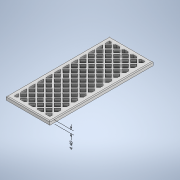
# Autodesk Inventor part: Part_B3
Saved by Autodesk Inventor 2022.6 (Build 266554010, 554A)
## iProperties
Created: 2025-05-15
Part Number: Part_B3
Material: Generic
Document SubType Name: Modeling
Designer: khinm
Density: 1 g/cm^3
Appearance: Default
Author: khinm
Autodesk Inventor part; units mm, degrees
ref_plane "YZ Plane" through (0, 0, 0) normal (1, 0, 0) x (0, 1, 0)
ref_plane "XZ Plane" through (0, 0, 0) normal (0, 1, 0) x (-1, 0, 0)
ref_plane "XY Plane" through (0, 0, 0) normal (0, 0, 1) x (1, 0, 0)
sketch "Sketch1" plane through (0, 0, 0) normal (0, 1, 0) x (-1, 0, 0)
  line L0 (27.35, -64.7) -> (-27.35, -64.7)
  line L1 (-27.35, -64.7) -> (-27.35, 64.7)
  line L2 (-27.35, 64.7) -> (27.35, 64.7)
  line L3 (27.35, 64.7) -> (27.35, -64.7)
  point P0 (0, 0)
  point P1 (27.35, 0)
  point P2 (0, -64.7)
  dimension "d0" = 54.7
  dimension "d1" = 129.4
  constraints: 8 end point, 2 midpoint, 2 parallel, 1 horizontal, 1 horizontal alignment, 1 perpendicular, 1 vertical alignment
  measures "d0" distance of L1.end L2.end
  measures "d1" distance between parallel lines of L2 L0
extrude "Extrusion1" add sketch "Sketch1" along normal mid plane 4.4
sketch "Sketch2" plane through (0, 2.2, 0) normal (0, 1, 0) x (1, 0, 0)
  line L0 (22.35, 59.7) -> (-22.35, 59.7)
  line L1 (-22.35, 59.7) -> (-22.35, -59.7)
  line L2 (-22.35, -59.7) -> (22.35, -59.7)
  line L3 (22.35, -59.7) -> (22.35, 59.7)
  line L4 (-27.35, -64.7) -> (27.35, -64.7) projected
  line L5 (-27.35, 64.7) -> (-27.35, -64.7) projected
  line L6 (-18.9137, 58.1363) -> (-22.35, 54.7)
  line L7 (21.949, -59.7) -> (22.35, -59.399)
  line L8 (-18.9137, -58.1363) -> (-22.35, -54.7)
  line L9 (21.899, 59.9) -> (22.4, 59.399)
  line L10 (16.3916, 58.1363) -> (19.8022, 54.7258)
  line L11 (21.6449, 53.033) -> (22.35, 52.328)
  line L12 (19.8772, 51.2652) -> (22.35, 48.7924)
  line L13 (22.35, 53.7381) -> (21.6449, 53.033)
  line L14 (17.9553, 59.7) -> (16.3916, 58.1363)
  line L15 (11.2924, 59.7) -> (12.8561, 58.1363)
  line L16 (14.6239, 56.5685) -> (18.1594, 53.033)
  line L17 (12.8561, 58.1363) -> (9.3206, 54.6008)
  line L18 (5.785, 58.1363) -> (9.3206, 54.6008)
  line L19 (14.6239, 56.5685) -> (11.0883, 53.033)
  line L20 (11.0883, 53.033) -> (14.6239, 49.4975)
  line L21 (9.3206, 51.2652) -> (12.8561, 47.7297)
  line L22 (19.8772, 51.2652) -> (16.3416, 47.7297)
  line L23 (16.3416, 47.7297) -> (19.8772, 44.1942)
  line L24 (21.6449, 42.4264) -> (22.35, 41.7214)
  line L25 (14.6239, 45.9619) -> (18.1594, 42.4264)
  line L26 (19.8772, 40.6586) -> (22.35, 38.1858)
  line L27 (22.35, 46.667) -> (19.8772, 44.1942)
  line L28 (22.35, 43.1315) -> (21.6449, 42.4264)
  line L29 (19.8772, 40.6586) -> (16.3416, 37.1231)
  line L30 (18.1594, 42.4264) -> (14.6239, 38.8909)
  line L31 (14.6239, 45.9619) -> (11.0883, 42.4264)
  line L32 (11.0883, 42.4264) -> (14.6239, 38.8909)
  line L33 (12.8561, 37.1231) -> (9.3206, 40.6586)
  line L34 (12.8561, 47.7297) -> (9.3206, 44.1942)
  line L35 (5.785, 47.7297) -> (9.3206, 44.1942)
  line L36 (9.3206, 51.2652) -> (5.785, 47.7297)
  line L37 (7.5528, 42.4264) -> (4.0173, 45.9619)
  line L38 (7.5528, 53.033) -> (4.0173, 49.4975)
  line L39 (16.3416, 37.1231) -> (19.8772, 33.5876)
  line L40 (21.6449, 31.8198) -> (22.35, 31.1148)
  line L41 (22.35, 27.5792) -> (19.8772, 30.052)
  line L42 (18.1594, 31.8198) -> (14.6239, 35.3553)
  line L43 (22.35, 32.5249) -> (21.6449, 31.8198)
  line L44 (22.35, 36.0604) -> (19.8772, 33.5876)
  line L45 (22.35, 20.5082) -> (21.6449, 21.2132)
  line L46 (22.35, 16.9726) -> (19.8772, 19.4454)
  line L47 (22.35, 21.9183) -> (21.6449, 21.2132)
  line L48 (22.35, 25.4538) -> (19.8772, 22.981)
  line L49 (19.8772, 30.052) -> (16.3416, 26.5165)
  line L50 (19.8772, 22.981) -> (16.3416, 26.5165)
  line L51 (18.1594, 21.2132) -> (14.6239, 24.7487)
  line L52 (18.1594, 31.8198) -> (14.6239, 28.2843)
  line L53 (14.6239, 35.3553) -> (11.0883, 31.8198)
  line L54 (12.8561, 37.1231) -> (9.3206, 33.5876)
  line L55 (9.3206, 40.6586) -> (5.785, 37.1231)
  line L56 (7.5528, 42.4264) -> (4.0173, 38.8909)
  line L57 (14.6239, 28.2843) -> (11.0883, 31.8198)
  line L58 (12.8561, 26.5165) -> (9.3206, 30.052)
  line L59 (9.3206, 22.981) -> (5.785, 26.5165)
  line L60 (7.5528, 21.2132) -> (4.0173, 24.7487)
  line L61 (14.6239, 17.6777) -> (11.0883, 21.2132)
  line L62 (12.8561, 15.9099) -> (9.3206, 19.4454)
  line L63 (9.3206, 12.3744) -> (5.785, 15.9099)
  line L64 (7.5528, 10.6066) -> (4.0173, 14.1421)
  line L65 (22.35, 9.9016) -> (21.6449, 10.6066)
  line L66 (19.8772, 12.3744) -> (16.3416, 15.9099)
  line L67 (22.35, 6.366) -> (19.8772, 8.8388)
  line L68 (18.1594, 10.6066) -> (14.6239, 14.1421)
  line L69 (14.6239, 7.0711) -> (11.0883, 10.6066)
  line L70 (12.8561, 5.3033) -> (9.3206, 8.8388)
  line L71 (22.35, 11.3117) -> (21.6449, 10.6066)
  line L72 (22.35, 14.8472) -> (19.8772, 12.3744)
  line L73 (19.8772, 19.4454) -> (16.3416, 15.9099)
  line L74 (18.1594, 21.2132) -> (14.6239, 17.6777)
  line L75 (14.6239, 24.7487) -> (11.0883, 21.2132)
  line L76 (12.8561, 26.5165) -> (9.3206, 22.981)
  line L77 (9.3206, 30.052) -> (5.785, 26.5165)
  line L78 (7.5528, 31.8198) -> (4.0173, 28.2843)
  line L79 (-18.9137, 58.1363) -> (-20.4774, 59.7)
  line L80 (-8.3571, 58.1363) -> (-9.9208, 59.7)
  line L81 (-11.8926, 54.6008) -> (-15.4282, 58.1363)
  line L82 (-13.6604, 53.033) -> (-17.1959, 56.5685)
  line L83 (-17.1959, 49.4975) -> (-20.7315, 53.033)
  line L84 (-18.9137, 47.5297) -> (-22.35, 50.966)
  line L85 (-3.2579, 59.7) -> (-4.8216, 58.1363)
  line L86 (-6.5893, 56.5685) -> (-10.1249, 53.033)
  line L87 (-8.3571, 58.1363) -> (-11.8926, 54.6008)
  line L88 (-13.8645, 59.7) -> (-15.4282, 58.1363)
  line L89 (-17.1959, 56.5685) -> (-20.7315, 53.033)
  line L90 (-11.8926, 51.2652) -> (-15.4282, 47.7297)
  line L91 (-17.1959, 45.9619) -> (-20.7315, 42.4264)
  line L92 (-13.6604, 53.033) -> (-17.1959, 49.4975)
  line L93 (-18.9137, 47.5297) -> (-22.35, 44.0934)
  line L94 (0.6858, 59.7) -> (2.2495, 58.1363)
  line L95 (4.0173, 56.5685) -> (7.5528, 53.033)
  line L96 (-4.8216, 58.1363) -> (-1.286, 54.6008)
  line L97 (0.4817, 53.033) -> (4.0173, 49.4975)
  line L98 (2.2495, 47.7297) -> (-1.286, 51.2652)
  line L99 (-3.0538, 53.033) -> (-6.5893, 56.5685)
  line L100 (-6.5893, 49.4975) -> (-10.1249, 53.033)
  line L101 (-8.3571, 47.7297) -> (-11.8926, 51.2652)
  line L102 (-11.8926, 44.1942) -> (-15.4282, 47.7297)
  line L103 (-13.6604, 42.4264) -> (-17.1959, 45.9619)
  line L104 (-17.1959, 38.8909) -> (-20.7315, 42.4264)
  line L105 (-18.9137, 36.9231) -> (-22.35, 40.3594)
  line L106 (7.3487, 59.7) -> (5.785, 58.1363)
  line L107 (4.0173, 56.5685) -> (0.4817, 53.033)
  line L108 (2.2495, 58.1363) -> (-1.286, 54.6008)
  line L109 (4.0173, 45.9619) -> (0.4817, 42.4264)
  line L110 (2.2495, 47.7297) -> (-1.286, 44.1942)
  line L111 (-1.286, 51.2652) -> (-4.8216, 47.7297)
  line L112 (-3.0538, 53.033) -> (-6.5893, 49.4975)
  line L113 (-1.286, 40.6586) -> (-4.8216, 37.1231)
  line L114 (-3.0538, 42.4264) -> (-6.5893, 38.8909)
  line L115 (-6.5893, 45.9619) -> (-10.1249, 42.4264)
  line L116 (-8.3571, 47.7297) -> (-11.8926, 44.1942)
  line L117 (-6.5893, 35.3553) -> (-10.1249, 31.8198)
  line L118 (-8.3571, 37.1231) -> (-11.8926, 33.5876)
  line L119 (-11.8926, 40.6586) -> (-15.4282, 37.1231)
  line L120 (-17.1959, 35.3553) -> (-20.7315, 31.8198)
  line L121 (-13.6604, 42.4264) -> (-17.1959, 38.8909)
  line L122 (-18.9137, 36.9231) -> (-22.35, 33.4868)
  line L123 (-11.8926, 30.052) -> (-15.4282, 26.5165)
  line L124 (-17.1959, 24.7487) -> (-20.7315, 21.2132)
  line L125 (-13.6604, 31.8198) -> (-17.1959, 28.2843)
  line L126 (-18.9137, 26.3165) -> (-22.35, 22.8802)
  line L127 (9.3206, 33.5876) -> (5.785, 37.1231)
  line L128 (7.5528, 31.8198) -> (4.0173, 35.3553)
  line L129 (4.0173, 28.2843) -> (0.4817, 31.8198)
  line L130 (2.2495, 26.5165) -> (-1.286, 30.052)
  line L131 (-17.1959, 17.6777) -> (-20.7315, 21.2132)
  line L132 (-18.9137, 15.7099) -> (-22.35, 19.1462)
  line L133 (4.0173, 35.3553) -> (0.4817, 31.8198)
  line L134 (2.2495, 37.1231) -> (-1.286, 33.5876)
  line L135 (-1.286, 30.052) -> (-4.8216, 26.5165)
  line L136 (-3.0538, 31.8198) -> (-6.5893, 28.2843)
  line L137 (-6.5893, 24.7487) -> (-10.1249, 21.2132)
  line L138 (-8.3571, 26.5165) -> (-11.8926, 22.981)
  line L139 (-11.8926, 19.4454) -> (-15.4282, 15.9099)
  line L140 (-17.1959, 14.1421) -> (-20.7315, 10.6066)
  line L141 (-13.6604, 21.2132) -> (-17.1959, 17.6777)
  line L142 (-18.9137, 15.7099) -> (-22.35, 12.2736)
  line L143 (4.0173, 17.6777) -> (0.4817, 21.2132)
  line L144 (-1.286, 22.981) -> (-4.8216, 26.5165)
  line L145 (2.2495, 15.9099) -> (-1.286, 19.4454)
  line L146 (-3.0538, 21.2132) -> (-6.5893, 24.7487)
  line L147 (-6.5893, 17.6777) -> (-10.1249, 21.2132)
  line L148 (-8.3571, 15.9099) -> (-11.8926, 19.4454)
  line L149 (-11.8926, 12.3744) -> (-15.4282, 15.9099)
  line L150 (-13.6604, 10.6066) -> (-17.1959, 14.1421)
  line L151 (-17.1959, 7.0711) -> (-20.7315, 10.6066)
  line L152 (-18.9137, 5.1033) -> (-22.35, 8.5396)
  line L153 (4.0173, 7.0711) -> (0.4817, 10.6066)
  line L154 (-1.286, 12.3744) -> (-4.8216, 15.9099)
  line L155 (2.2495, 5.3033) -> (-1.286, 8.8388)
  line L156 (-3.0538, 10.6066) -> (-6.5893, 14.1421)
  line L157 (-6.5893, 7.0711) -> (-10.1249, 10.6066)
  line L158 (-8.3571, 5.3033) -> (-11.8926, 8.8388)
  line L159 (-11.8926, 1.7678) -> (-15.4282, 5.3033)
  line L160 (-13.6604, 0) -> (-17.1959, 3.5355)
  line L161 (-17.1959, -3.5355) -> (-20.7315, 0)
  line L162 (-18.9137, -5.5033) -> (-22.35, -2.067)
  line L163 (-1.286, 1.7678) -> (-4.8216, 5.3033)
  line L164 (-3.0538, 0) -> (-6.5893, 3.5355)
  line L165 (-6.5893, -3.5355) -> (-10.1249, 0)
  line L166 (-8.3571, -5.3033) -> (-11.8926, -1.7678)
  line L167 (-11.8926, -8.8388) -> (-15.4282, -5.3033)
  line L168 (-13.6604, -10.6066) -> (-17.1959, -7.0711)
  line L169 (-17.1959, -14.1421) -> (-20.7315, -10.6066)
  line L170 (-18.9137, -16.1099) -> (-22.35, -12.6736)
  line L171 (9.3206, 1.7678) -> (5.785, 5.3033)
  line L172 (7.5528, 0) -> (4.0173, 3.5355)
  line L173 (4.0173, -3.5355) -> (0.4817, 0)
  line L174 (2.2495, -5.3033) -> (-1.286, -1.7678)
  line L175 (-1.286, -8.8388) -> (-4.8216, -5.3033)
  line L176 (-3.0538, -10.6066) -> (-6.5893, -7.0711)
  line L177 (-6.5893, -14.1421) -> (-10.1249, -10.6066)
  line L178 (-8.3571, -15.9099) -> (-11.8926, -12.3744)
  line L179 (-11.8926, -19.4454) -> (-15.4282, -15.9099)
  line L180 (-13.6604, -21.2132) -> (-17.1959, -17.6777)
  line L181 (-17.1959, -24.7487) -> (-20.7315, -21.2132)
  line L182 (-18.9137, -26.7165) -> (-22.35, -23.2802)
  line L183 (-18.9137, -37.3231) -> (-22.35, -33.8868)
  line L184 (-17.1959, -35.3553) -> (-20.7315, -31.8198)
  line L185 (-13.6604, -31.8198) -> (-17.1959, -28.2843)
  line L186 (-11.8926, -30.052) -> (-15.4282, -26.5165)
  line L187 (-8.3571, -26.5165) -> (-11.8926, -22.981)
  line L188 (-6.5893, -24.7487) -> (-10.1249, -21.2132)
  line L189 (-3.0538, -21.2132) -> (-6.5893, -17.6777)
  line L190 (-1.286, -19.4454) -> (-4.8216, -15.9099)
  line L191 (2.2495, -15.9099) -> (-1.286, -12.3744)
  line L192 (4.0173, -14.1421) -> (0.4817, -10.6066)
  line L193 (7.5528, -10.6066) -> (4.0173, -7.0711)
  line L194 (9.3206, -8.8388) -> (5.785, -5.3033)
  line L195 (22.35, -0.7051) -> (21.6449, 0)
  line L196 (19.8772, 1.7678) -> (16.3416, 5.3033)
  line L197 (22.35, 0) -> (21.6449, 0)
  line L198 (22.35, -4.2406) -> (19.8772, -1.7678)
  line L199 (18.1594, 0) -> (14.6239, 3.5355)
  line L200 (14.6239, -3.5355) -> (11.0883, 0)
  line L201 (12.8561, -5.3033) -> (9.3206, -1.7678)
  line L202 (22.35, -11.3117) -> (21.6449, -10.6066)
  line L203 (19.8772, -8.8388) -> (16.3416, -5.3033)
  line L204 (22.35, -14.8472) -> (19.8772, -12.3744)
  line L205 (18.1594, -10.6066) -> (14.6239, -7.0711)
  line L206 (14.6239, -14.1421) -> (11.0883, -10.6066)
  line L207 (12.8561, -15.9099) -> (9.3206, -12.3744)
  line L208 (9.3206, -19.4454) -> (5.785, -15.9099)
  line L209 (7.5528, -21.2132) -> (4.0173, -17.6777)
  line L210 (4.0173, -24.7487) -> (0.4817, -21.2132)
  line L211 (2.2495, -26.5165) -> (-1.286, -22.981)
  line L212 (-1.286, -30.052) -> (-4.8216, -26.5165)
  line L213 (-3.0538, -31.8198) -> (-6.5893, -28.2843)
  line L214 (-6.5893, -35.3553) -> (-10.1249, -31.8198)
  line L215 (-8.3571, -37.1231) -> (-11.8926, -33.5876)
  line L216 (-11.8926, -40.6586) -> (-15.4282, -37.1231)
  line L217 (-13.6604, -42.4264) -> (-17.1959, -38.8909)
  line L218 (-17.1959, -45.9619) -> (-20.7315, -42.4264)
  line L219 (-18.9137, -47.9297) -> (-22.35, -44.4934)
  line L220 (22.35, -21.9183) -> (21.6449, -21.2132)
  line L221 (19.8772, -19.4454) -> (16.3416, -15.9099)
  line L222 (22.35, -25.4538) -> (19.8772, -22.981)
  line L223 (18.1594, -21.2132) -> (14.6239, -17.6777)
  line L224 (14.6239, -24.7487) -> (11.0883, -21.2132)
  line L225 (12.8561, -26.5165) -> (9.3206, -22.981)
  line L226 (9.3206, -30.052) -> (5.785, -26.5165)
  line L227 (7.5528, -31.8198) -> (4.0173, -28.2843)
  line L228 (4.0173, -35.3553) -> (0.4817, -31.8198)
  line L229 (2.2495, -37.1231) -> (-1.286, -33.5876)
  line L230 (-1.286, -40.6586) -> (-4.8216, -37.1231)
  line L231 (-3.0538, -42.4264) -> (-6.5893, -38.8909)
  line L232 (-6.5893, -45.9619) -> (-10.1249, -42.4264)
  line L233 (-8.3571, -47.7297) -> (-11.8926, -44.1942)
  line L234 (-11.8926, -51.2652) -> (-15.4282, -47.7297)
  line L235 (-8.3071, -58.1363) -> (-11.8426, -54.6008)
  line L236 (-13.6604, -53.033) -> (-17.1959, -49.4975)
  line L237 (-13.8145, -59.7) -> (-15.3782, -58.1363)
  line L238 (-17.1959, -56.5685) -> (-20.7315, -53.033)
  line L239 (22.35, -32.5249) -> (21.6449, -31.8198)
  line L240 (19.8772, -30.052) -> (16.3416, -26.5165)
  line L241 (22.35, -36.0604) -> (19.8772, -33.5876)
  line L242 (18.1594, -31.8198) -> (14.6239, -28.2843)
  line L243 (14.6239, -35.3553) -> (11.0883, -31.8198)
  line L244 (12.8561, -37.1231) -> (9.3206, -33.5876)
  line L245 (9.3206, -40.6586) -> (5.785, -37.1231)
  line L246 (7.5528, -42.4264) -> (4.0173, -38.8909)
  line L247 (4.0173, -45.9619) -> (0.4817, -42.4264)
  line L248 (2.2495, -47.7297) -> (-1.286, -44.1942)
  line L249 (-1.286, -51.2652) -> (-4.8216, -47.7297)
  line L250 (2.2995, -58.1363) -> (-1.236, -54.6008)
  line L251 (-3.0538, -53.033) -> (-6.5893, -49.4975)
  line L252 (-3.2079, -59.7) -> (-4.7716, -58.1363)
  line L253 (-6.5893, -56.5685) -> (-10.1249, -53.033)
  line L254 (22.35, -43.1315) -> (21.6449, -42.4264)
  line L255 (19.8772, -40.6586) -> (16.3416, -37.1231)
  line L256 (22.35, -46.667) -> (19.8772, -44.1942)
  line L257 (18.1594, -42.4264) -> (14.6239, -38.8909)
  line L258 (14.6239, -45.9619) -> (11.0883, -42.4264)
  line L259 (12.8561, -47.7297) -> (9.3206, -44.1942)
  line L260 (9.3206, -51.2652) -> (5.785, -47.7297)
  line L261 (12.9061, -58.1363) -> (9.3706, -54.6008)
  line L262 (7.5528, -53.033) -> (4.0173, -49.4975)
  line L263 (7.3987, -59.7) -> (5.835, -58.1363)
  line L264 (4.0173, -56.5685) -> (0.4817, -53.033)
  line L265 (22.35, -53.7381) -> (21.6449, -53.033)
  line L266 (19.8772, -51.2652) -> (16.3416, -47.7297)
  line L267 (22.4, -57.2736) -> (19.9272, -54.8008)
  line L268 (18.1594, -53.033) -> (14.6239, -49.4975)
  line L269 (17.9553, -59.9) -> (16.3916, -58.3363)
  line L270 (14.6239, -56.5685) -> (11.0883, -53.033)
  line L271 (-18.9137, -58.1363) -> (-20.4774, -59.7)
  line L272 (-8.3071, -58.1363) -> (-9.8708, -59.7)
  line L273 (-11.8426, -54.6008) -> (-15.3782, -58.1363)
  line L274 (-13.6604, -53.033) -> (-17.1959, -56.5685)
  line L275 (-17.1959, -49.4975) -> (-20.7315, -53.033)
  line L276 (-18.9137, -47.9297) -> (-22.35, -51.366)
  line L277 (0.7358, -59.7) -> (2.2995, -58.1363)
  line L278 (-4.7716, -58.1363) -> (-1.236, -54.6008)
  line L279 (-3.0538, -53.033) -> (-6.5893, -56.5685)
  line L280 (-6.5893, -49.4975) -> (-10.1249, -53.033)
  line L281 (-8.3571, -47.7297) -> (-11.8926, -51.2652)
  line L282 (-11.8926, -44.1942) -> (-15.4282, -47.7297)
  line L283 (-13.6604, -42.4264) -> (-17.1959, -45.9619)
  line L284 (-17.1959, -38.8909) -> (-20.7315, -42.4264)
  line L285 (-18.9137, -37.3231) -> (-22.35, -40.7594)
  line L286 (11.3424, -59.7) -> (12.9061, -58.1363)
  line L287 (5.835, -58.1363) -> (9.3706, -54.6008)
  line L288 (4.0173, -56.5685) -> (7.5528, -53.033)
  line L289 (0.4817, -53.033) -> (4.0173, -49.4975)
  line L290 (2.2495, -47.7297) -> (-1.286, -51.2652)
  line L291 (-1.286, -44.1942) -> (-4.8216, -47.7297)
  line L292 (-3.0538, -42.4264) -> (-6.5893, -45.9619)
  line L293 (-6.5893, -38.8909) -> (-10.1249, -42.4264)
  line L294 (-8.3571, -37.1231) -> (-11.8926, -40.6586)
  line L295 (-11.8926, -33.5876) -> (-15.4282, -37.1231)
  line L296 (-13.6604, -31.8198) -> (-17.1959, -35.3553)
  line L297 (-17.1959, -28.2843) -> (-20.7315, -31.8198)
  line L298 (-18.9137, -26.7165) -> (-22.35, -30.1528)
  line L299 (-18.9137, -16.1099) -> (-22.35, -19.5462)
  line L300 (-17.1959, -17.6777) -> (-20.7315, -21.2132)
  line L301 (-13.6604, -21.2132) -> (-17.1959, -24.7487)
  line L302 (-11.8926, -22.981) -> (-15.4282, -26.5165)
  line L303 (-8.3571, -26.5165) -> (-11.8926, -30.052)
  line L304 (-6.5893, -28.2843) -> (-10.1249, -31.8198)
  line L305 (-3.0538, -31.8198) -> (-6.5893, -35.3553)
  line L306 (-1.286, -33.5876) -> (-4.8216, -37.1231)
  line L307 (2.2495, -37.1231) -> (-1.286, -40.6586)
  line L308 (4.0173, -38.8909) -> (0.4817, -42.4264)
  line L309 (7.5528, -42.4264) -> (4.0173, -45.9619)
  line L310 (5.785, -47.7297) -> (9.3206, -44.1942)
  line L311 (9.3206, -51.2652) -> (12.8561, -47.7297)
  line L312 (11.0883, -53.033) -> (14.6239, -49.4975)
  line L313 (14.6239, -56.5685) -> (18.1594, -53.033)
  line L314 (19.8772, -51.2652) -> (22.35, -48.7924)
  line L315 (16.3916, -58.3363) -> (19.9272, -54.8008)
  line L316 (21.6449, -53.033) -> (22.35, -52.328)
  line L317 (-18.9137, -5.5033) -> (-22.35, -8.9396)
  line L318 (-17.1959, -7.0711) -> (-20.7315, -10.6066)
  line L319 (-13.6604, -10.6066) -> (-17.1959, -14.1421)
  line L320 (-11.8926, -12.3744) -> (-15.4282, -15.9099)
  line L321 (-8.3571, -15.9099) -> (-11.8926, -19.4454)
  line L322 (-6.5893, -17.6777) -> (-10.1249, -21.2132)
  line L323 (-3.0538, -21.2132) -> (-6.5893, -24.7487)
  line L324 (-1.286, -22.981) -> (-4.8216, -26.5165)
  line L325 (2.2495, -26.5165) -> (-1.286, -30.052)
  line L326 (4.0173, -28.2843) -> (0.4817, -31.8198)
  line L327 (7.5528, -31.8198) -> (4.0173, -35.3553)
  line L328 (9.3206, -33.5876) -> (5.785, -37.1231)
  line L329 (12.8561, -37.1231) -> (9.3206, -40.6586)
  line L330 (11.0883, -42.4264) -> (14.6239, -38.8909)
  line L331 (14.6239, -45.9619) -> (18.1594, -42.4264)
  line L332 (19.8772, -40.6586) -> (22.35, -38.1858)
  line L333 (16.3416, -47.7297) -> (19.8772, -44.1942)
  line L334 (21.6449, -42.4264) -> (22.35, -41.7214)
  line L335 (-18.9137, 5.1033) -> (-22.35, 1.667)
  line L336 (-17.1959, 3.5355) -> (-20.7315, 0)
  line L337 (-13.6604, 0) -> (-17.1959, -3.5355)
  line L338 (-11.8926, -1.7678) -> (-15.4282, -5.3033)
  line L339 (-8.3571, -5.3033) -> (-11.8926, -8.8388)
  line L340 (-6.5893, -7.0711) -> (-10.1249, -10.6066)
  line L341 (-3.0538, -10.6066) -> (-6.5893, -14.1421)
  line L342 (-1.286, -12.3744) -> (-4.8216, -15.9099)
  line L343 (2.2495, -15.9099) -> (-1.286, -19.4454)
  line L344 (4.0173, -17.6777) -> (0.4817, -21.2132)
  line L345 (7.5528, -21.2132) -> (4.0173, -24.7487)
  line L346 (9.3206, -22.981) -> (5.785, -26.5165)
  line L347 (12.8561, -26.5165) -> (9.3206, -30.052)
  line L348 (14.6239, -28.2843) -> (11.0883, -31.8198)
  line L349 (22.35, -27.5792) -> (19.8772, -30.052)
  line L350 (18.1594, -31.8198) -> (14.6239, -35.3553)
  line L351 (16.3416, -37.1231) -> (19.8772, -33.5876)
  line L352 (21.6449, -31.8198) -> (22.35, -31.1148)
  line L353 (-13.6604, 10.6066) -> (-17.1959, 7.0711)
  line L354 (-11.8926, 8.8388) -> (-15.4282, 5.3033)
  line L355 (-8.3571, 5.3033) -> (-11.8926, 1.7678)
  line L356 (-6.5893, 3.5355) -> (-10.1249, 0)
  line L357 (-3.0538, 0) -> (-6.5893, -3.5355)
  line L358 (-1.286, -1.7678) -> (-4.8216, -5.3033)
  line L359 (2.2495, -5.3033) -> (-1.286, -8.8388)
  line L360 (4.0173, -7.0711) -> (0.4817, -10.6066)
  line L361 (7.5528, -10.6066) -> (4.0173, -14.1421)
  line L362 (9.3206, -12.3744) -> (5.785, -15.9099)
  line L363 (12.8561, -15.9099) -> (9.3206, -19.4454)
  line L364 (14.6239, -17.6777) -> (11.0883, -21.2132)
  line L365 (22.35, -16.9726) -> (19.8772, -19.4454)
  line L366 (18.1594, -21.2132) -> (14.6239, -24.7487)
  line L367 (22.35, -20.5082) -> (21.6449, -21.2132)
  line L368 (19.8772, -22.981) -> (16.3416, -26.5165)
  line L369 (-8.3571, 15.9099) -> (-11.8926, 12.3744)
  line L370 (-6.5893, 14.1421) -> (-10.1249, 10.6066)
  line L371 (-3.0538, 10.6066) -> (-6.5893, 7.0711)
  line L372 (-1.286, 8.8388) -> (-4.8216, 5.3033)
  line L373 (2.2495, 5.3033) -> (-1.286, 1.7678)
  line L374 (4.0173, 3.5355) -> (0.4817, 0)
  line L375 (7.5528, 0) -> (4.0173, -3.5355)
  line L376 (9.3206, -1.7678) -> (5.785, -5.3033)
  line L377 (12.8561, -5.3033) -> (9.3206, -8.8388)
  line L378 (14.6239, -7.0711) -> (11.0883, -10.6066)
  line L379 (22.35, -6.366) -> (19.8772, -8.8388)
  line L380 (18.1594, -10.6066) -> (14.6239, -14.1421)
  line L381 (22.35, -9.9016) -> (21.6449, -10.6066)
  line L382 (19.8772, -12.3744) -> (16.3416, -15.9099)
  line L383 (2.2495, 26.5165) -> (-1.286, 22.981)
  line L384 (-3.0538, 21.2132) -> (-6.5893, 17.6777)
  line L385 (4.0173, 24.7487) -> (0.4817, 21.2132)
  line L386 (-1.286, 19.4454) -> (-4.8216, 15.9099)
  line L387 (7.5528, 21.2132) -> (4.0173, 17.6777)
  line L388 (2.2495, 15.9099) -> (-1.286, 12.3744)
  line L389 (9.3206, 19.4454) -> (5.785, 15.9099)
  line L390 (4.0173, 14.1421) -> (0.4817, 10.6066)
  line L391 (12.8561, 15.9099) -> (9.3206, 12.3744)
  line L392 (7.5528, 10.6066) -> (4.0173, 7.0711)
  line L393 (14.6239, 14.1421) -> (11.0883, 10.6066)
  line L394 (9.3206, 8.8388) -> (5.785, 5.3033)
  line L395 (18.1594, 10.6066) -> (14.6239, 7.0711)
  line L396 (12.8561, 5.3033) -> (9.3206, 1.7678)
  line L397 (19.8772, 8.8388) -> (16.3416, 5.3033)
  line L398 (14.6239, 3.5355) -> (11.0883, 0)
  line L399 (22.35, 4.2406) -> (19.8772, 1.7678)
  line L400 (18.1594, 0) -> (14.6239, -3.5355)
  line L401 (22.35, 0.7051) -> (21.6449, 0)
  line L402 (19.8772, -1.7678) -> (16.3416, -5.3033)
  line L403 (22.35, 57.2736) -> (19.8022, 54.7258)
  line L404 (18.1594, 53.033) -> (14.6239, 49.4975)
  line L405 (4.0173, 38.8909) -> (0.4817, 42.4264)
  line L406 (-1.286, 44.1942) -> (-4.8216, 47.7297)
  line L407 (2.2495, 37.1231) -> (-1.286, 40.6586)
  line L408 (-3.0538, 42.4264) -> (-6.5893, 45.9619)
  line L409 (-1.286, 33.5876) -> (-4.8216, 37.1231)
  line L410 (-6.5893, 38.8909) -> (-10.1249, 42.4264)
  line L411 (-3.0538, 31.8198) -> (-6.5893, 35.3553)
  line L412 (-8.3571, 37.1231) -> (-11.8926, 40.6586)
  line L413 (-6.5893, 28.2843) -> (-10.1249, 31.8198)
  line L414 (-11.8926, 33.5876) -> (-15.4282, 37.1231)
  line L415 (-8.3571, 26.5165) -> (-11.8926, 30.052)
  line L416 (-13.6604, 31.8198) -> (-17.1959, 35.3553)
  line L417 (-11.8926, 22.981) -> (-15.4282, 26.5165)
  line L418 (-17.1959, 28.2843) -> (-20.7315, 31.8198)
  line L419 (-13.6604, 21.2132) -> (-17.1959, 24.7487)
  line L420 (-18.9137, 26.3165) -> (-22.35, 29.7528)
  point P0 (0, 0)
  point P1 (0, -59.7)
  point P2 (-22.35, 51.1645)
  point P3 (-6.7934, 59.7)
  point P4 (-22.35, 40.5579)
  point P5 (3.8132, 59.7)
  point P6 (-22.35, 29.9513)
  point P7 (-22.35, 8.7381)
  point P8 (-22.4, 1.6685)
  point P9 (-22.4, 12.2751)
  point P10 (-22.4, 33.4883)
  point P11 (-22.4, 44.0949)
  point P12 (-22.4, 54.7016)
  point P13 (-16.9918, 59.9)
  point P14 (-6.3852, 59.9)
  point P15 (14.828, 59.9)
  point P16 (4.2214, 59.9)
  point P17 (-13.8145, -59.7)
  point P18 (-3.2079, -59.7)
  point P19 (-22.35, -54.7)
  point P20 (-22.35, -44.4934)
  point P21 (-22.35, -33.8868)
  point P22 (-22.35, -23.2802)
  point P23 (-22.35, -12.6736)
  point P24 (-22.35, -2.067)
  point P25 (-22.35, 8.5396)
  point P26 (-22.35, 19.1462)
  point P27 (-22.35, 29.7528)
  point P28 (-22.35, 40.3594)
  point P29 (-22.35, 50.966)
  point P30 (-20.4774, 59.7)
  point P31 (-9.9208, 59.7)
  point P32 (0.6858, 59.7)
  point P33 (7.3987, -59.7)
  point P34 (17.7553, -59.7)
  point P35 (22.35, -57.2236)
  point P36 (22.35, -46.667)
  point P37 (22.35, -36.0604)
  point P38 (22.35, -25.4538)
  point P39 (22.35, -14.8472)
  point P40 (22.35, -4.2406)
  point P41 (22.35, 6.366)
  point P42 (22.35, 16.9726)
  point P43 (22.35, 27.5792)
  point P44 (22.35, 38.1858)
  point P45 (22.35, 48.7924)
  point P46 (11.2924, 59.7)
  point P47 (22.35, 59.449)
  point P48 (22.099, 59.7)
  dimension "d4" = 5
  dimension "d5" = 5
  dimension "d6" = 5
  dimension "d44" = 1.8726
  constraints: 1503 parallel, 834 end point, 11 point on line, 2 horizontal, 1 horizontal alignment, 1 midpoint, 1 vertical alignment, 45 other
  measures "d4" distance between parallel lines of L4 L2
  measures "d6" distance of L6.end L0.end
  measures "d44" distance of L0.end L79.end
extrude "Extrusion2" cut sketch "Sketch2" against normal up to surface (4.4 mm away) contours L0 L9 L3 L403 L10 L14 | L15 L17 L18 L106 L0 | L94 L108 L96 L85 L0 | L80 L87 L81 L88 L0 | L3 L27 L23 L22 L12 | L79 L6 L1 L0 | L84 L93 L1 | L3 L44 L39 L29 L26 | L105 L122 L1 | L420 L126 L1 | L3 L48 L50 L49 L41 | L132 L142 L1 | L152 L335 L1 | L3 L72 L66 L73 L46 | L162 L317 L1 | L170 L299 L1 | L3 L399 L196 L397 L67 | L182 L298 L1 | L183 L285 L1 | L3 L379 L203 L402 L198 | L219 L276 L1 | L8 L271 L2 L1 | L3 L365 L221 L382 L204 | L237 L273 L235 L272 L2 | L252 L278 L250 L277 L2 | L3 L349 L240 L368 L222 | L263 L287 L261 L286 L2 | L269 L315 L267 L3 L7 L2 | L3 L332 L255 L351 L241 | L3 L314 L266 L333 L256 | L16 L404 L20 L19 | L21 L34 L35 L36 | L25 L30 L32 L31 | L54 L127 L55 L33 | L56 L405 L109 L37 | L38 L97 L107 L95 | L52 L57 L53 L42 | L74 L61 L75 L51 | L76 L59 L77 L58 | L387 L143 L385 L60 | L391 L63 L389 L62 | L392 L153 L390 L64 | L395 L69 L393 L68 | L396 L171 L394 L70 | L78 L129 L133 L128 | L92 L83 L89 L82 | L99 L112 L100 L86 | L101 L116 L102 L90 | L103 L121 L104 L91 | L110 L406 L111 L98 | L407 L134 L409 L113 | L114 L410 L115 L408 | L411 L136 L413 L117 | L118 L414 L119 L412 | L416 L125 L418 L120 | L415 L138 L417 L123 | L419 L141 L131 L124 | L383 L144 L135 L130 | L146 L384 L147 L137 | L148 L369 L149 L139 | L150 L353 L151 L140 | L388 L154 L386 L145 | L373 L163 L372 L155 | L371 L157 L370 L156 | L355 L159 L354 L158 | L337 L161 L336 L160 | L357 L165 L356 L164 | L339 L167 L338 L166 | L319 L169 L318 L168 | L375 L173 L374 L172 | L359 L175 L358 L174 | L341 L177 L340 L176 | L321 L179 L320 L178 | L301 L181 L300 L180 | L184 L297 L185 L296 | L186 L302 L187 L303 | L188 L322 L189 L323 | L190 L342 L191 L343 | L192 L360 L193 L361 | L194 L376 L201 L377 | L400 L200 L398 L199 | L380 L206 L378 L205 | L363 L208 L362 L207 | L345 L210 L344 L209 | L325 L212 L324 L211 | L305 L214 L304 L213 | L294 L216 L295 L215 | L283 L218 L284 L217 | L366 L224 L364 L223 | L347 L226 L346 L225 | L327 L228 L326 L227 | L307 L230 L306 L229 | L292 L232 L293 L231 | L281 L234 L282 L233 | L274 L238 L275 L236 | L350 L243 L348 L242 | L329 L245 L328 L244 | L309 L247 L308 L246 | L290 L249 L291 L248 | L279 L253 L280 L251 | L331 L258 L330 L257 | L311 L260 L310 L259 | L288 L264 L289 L262 | L313 L270 L312 L268
chamfer "Chamfer1" distance 0.4 angle 45 379 edges at (-20.6318, 2.2, 56.4182) (-19.6955, 2.2, 58.9182) (-18.9637, 2.2, 54.8008) (-20.6318, 2.2, 49.6479) (-18.9637, 2.2, 51.2652) (-13.6104, 2.2, 56.3685) (-15.4282, 2.2, 54.8008) (-10.1249, 2.2, 49.4975) (-8.3571, 2.2, 51.2652) (-13.6604, 2.2, 45.9619) (-15.4282, 2.2, 44.1942) (-18.9637, 2.2, 40.6586) (-20.6318, 2.2, 39.0413) (-15.4282, 2.2, 33.5876) (-13.6604, 2.2, 35.3553) (-18.9637, 2.2, 44.1942) (-20.6318, 2.2, 46.2116) (-15.4282, 2.2, 51.2652) (-13.6604, 2.2, 49.4975) (-10.0749, 2.2, 56.3685) (-8.3571, 2.2, 54.8008) (-4.8216, 2.2, 54.8008) (-14.5963, 2.2, 58.9182) (-4.8216, 2.2, 51.2652) (-8.3571, 2.2, 44.1942) (-10.1249, 2.2, 45.9619) (-13.6604, 2.2, 38.8909) (-15.4282, 2.2, 40.6586) (-18.9637, 2.2, 33.5876) (-20.6318, 2.2, 35.605) (-20.6318, 2.2, 28.4347) (-18.9637, 2.2, 30.052) (-20.6318, 2.2, 24.9983) (-18.9637, 2.2, 22.981) (-13.6604, 2.2, 28.2843) (-15.4282, 2.2, 30.052) (-10.1249, 2.2, 35.3553) (-8.3571, 2.2, 33.5876) (-4.8216, 2.2, 40.6586) (-3.0538, 2.2, 38.8909) (-8.3571, 2.2, 40.6586) (-4.8216, 2.2, 44.1942) (-3.0538, 2.2, 45.9619) (-3.0538, 2.2, 49.4975) (0.4817, 2.2, 49.4975) (2.2495, 2.2, 51.2652) (5.785, 2.2, 54.8008) (2.2495, 2.2, 54.8008) (5.785, 2.2, 51.2652) (0.5317, 2.2, 56.3685) (-3.0038, 2.2, 56.3685) (-3.9897, 2.2, 58.9182) (1.5177, 2.2, 58.9182) (6.6169, 2.2, 58.9182) (7.6028, 2.2, 56.3685) (11.1383, 2.2, 56.3685) (12.1243, 2.2, 58.9182) (12.8561, 2.2, 54.8008) (12.8561, 2.2, 51.2652) (16.3916, 2.2, 54.8008) (16.3916, 2.2, 51.2652) (21.1386, 2.2, 56.0122) (18.1594, 2.2, 56.5685) (17.0735, 2.2, 59.0182) (18.1094, 2.2, 49.4975) (18.1094, 2.2, 45.9619) (21.1136, 2.2, 50.0288) (21.1136, 2.2, 45.4306) (12.8561, 2.2, 44.1942) (12.8561, 2.2, 40.6586) (16.3916, 2.2, 40.6586) (16.3916, 2.2, 44.1942) (11.0883, 2.2, 45.9619) (7.5528, 2.2, 45.9619) (11.0883, 2.2, 49.4975) (7.5528, 2.2, 49.4975) (5.785, 2.2, 44.1942) (2.2495, 2.2, 40.6586) (5.785, 2.2, 40.6586) (2.2495, 2.2, 44.1942) (0.4817, 2.2, 38.8909) (-3.0538, 2.2, 35.3553) (0.4817, 2.2, 35.3553) (-4.8216, 2.2, 33.5876) (-8.3571, 2.2, 30.052) (-4.8216, 2.2, 30.052) (-10.1249, 2.2, 28.2843) (-13.6604, 2.2, 24.7487) (-15.4282, 2.2, 22.981) (-18.9637, 2.2, 19.4454) (-20.6318, 2.2, 17.8281) (-20.6318, 2.2, 14.3917) (-18.9637, 2.2, 8.8388) (-18.9637, 2.2, 12.3744) (-15.4282, 2.2, 8.8388) (-20.6318, 2.2, 7.2215) (-20.6318, 2.2, 3.7851) (-15.4282, 2.2, 1.7678) (-10.1249, 2.2, 7.0711) (-13.6604, 2.2, 3.5355) (-18.9637, 2.2, -1.7678) (-18.9637, 2.2, 1.7678) (-10.1249, 2.2, 14.1421) (-13.6604, 2.2, 14.1421) (-13.6604, 2.2, 17.6777) (-10.1249, 2.2, 17.6777) (-8.3571, 2.2, 19.4454) (-4.8216, 2.2, 22.981) (-4.8216, 2.2, 19.4454) (-8.3571, 2.2, 22.981) (-3.0538, 2.2, 24.7487) (0.4817, 2.2, 28.2843) (2.2495, 2.2, 30.052) (5.785, 2.2, 33.5876) (5.785, 2.2, 30.052) (2.2495, 2.2, 33.5876) (-3.0538, 2.2, 28.2843) (0.4817, 2.2, 24.7487) (7.5528, 2.2, 35.3553) (11.0883, 2.2, 35.3553) (11.0883, 2.2, 38.8909) (7.5528, 2.2, 38.8909) (18.1094, 2.2, 38.8909) (18.1094, 2.2, 35.3553) (21.1136, 2.2, 39.4222) (21.1136, 2.2, 34.824) (16.3916, 2.2, 33.5876) (12.8561, 2.2, 30.052) (16.3916, 2.2, 30.052) (12.8561, 2.2, 33.5876) (11.0883, 2.2, 28.2843) (7.5528, 2.2, 24.7487) (11.0883, 2.2, 24.7487) (7.5528, 2.2, 28.2843) (5.785, 2.2, 22.981) (5.785, 2.2, 19.4454) (2.2495, 2.2, 19.4454) (2.2495, 2.2, 22.981) (0.4817, 2.2, 17.6777) (-3.0538, 2.2, 14.1421) (0.4817, 2.2, 14.1421) (-3.0538, 2.2, 17.6777) (-8.3571, 2.2, 8.8388) (-4.8216, 2.2, 8.8388) (-4.8216, 2.2, 12.3744) (-8.3571, 2.2, 12.3744) (-10.1249, 2.2, -3.5355) (-13.6604, 2.2, -7.0711) (-13.6604, 2.2, -3.5355) (-15.4282, 2.2, -1.7678) (-10.1249, 2.2, -7.0711) (-4.8216, 2.2, 1.7678) (-8.3571, 2.2, -1.7678) (-4.8216, 2.2, -1.7678) (-8.3571, 2.2, 1.7678) (-3.0538, 2.2, 3.5355) (0.4817, 2.2, 7.0711) (0.4817, 2.2, 3.5355) (-3.0538, 2.2, 7.0711) (2.2495, 2.2, 8.8388) (5.785, 2.2, 12.3744) (5.785, 2.2, 8.8388) (2.2495, 2.2, 12.3744) (7.5528, 2.2, 14.1421) (11.0883, 2.2, 17.6777) (11.0883, 2.2, 14.1421) (7.5528, 2.2, 17.6777) (16.3916, 2.2, 22.981) (12.8561, 2.2, 19.4454) (16.3916, 2.2, 19.4454) (12.8561, 2.2, 22.981) (18.1094, 2.2, 24.7487) (21.1136, 2.2, 28.8156) (21.1136, 2.2, 24.2174) (18.1094, 2.2, 28.2843) (18.1094, 2.2, 17.6777) (18.1094, 2.2, 14.1421) (21.1136, 2.2, 18.209) (21.1136, 2.2, 13.6108) (12.8561, 2.2, 8.8388) (16.3916, 2.2, 12.3744) (12.8561, 2.2, 12.3744) (16.3916, 2.2, 8.8388) (7.5528, 2.2, 3.5355) (11.0883, 2.2, 7.0711) (7.5528, 2.2, 7.0711) (11.0883, 2.2, 3.5355) (5.785, 2.2, 1.7678) (2.2495, 2.2, -1.7678) (5.785, 2.2, -1.7678) (2.2495, 2.2, 1.7678) (0.4817, 2.2, -3.5355) (-3.0538, 2.2, -7.0711) (-3.0538, 2.2, -3.5355) (0.4817, 2.2, -7.0711) (18.1094, 2.2, 3.5355) (18.1094, 2.2, 7.0711) (-15.4282, 2.2, -12.3744) (-18.9637, 2.2, -12.3744) (-18.9637, 2.2, -8.8388) (-15.4282, 2.2, -8.8388) (-20.6318, 2.2, -6.8215) (-20.6318, 2.2, -3.3851) (-20.6318, 2.2, -13.9917) (-20.6318, 2.2, -17.4281) (-18.9637, 2.2, -19.4454) (-18.9637, 2.2, -22.981) (-20.6318, 2.2, -24.5983) (-20.6318, 2.2, -28.0347) (-18.9637, 2.2, -30.052) (-15.4282, 2.2, -30.052) (-13.6604, 2.2, -28.2843) (-13.6604, 2.2, -24.7487) (-15.4282, 2.2, -22.981) (-10.1249, 2.2, -24.7487) (-8.3571, 2.2, -22.981) (-4.8216, 2.2, -19.4454) (-3.0538, 2.2, -17.6777) (0.4817, 2.2, -14.1421) (2.2495, 2.2, -12.3744) (5.785, 2.2, -8.8388) (7.5528, 2.2, -7.0711) (11.0883, 2.2, -3.5355) (12.8561, 2.2, -1.7678) (16.3916, 2.2, 1.7678) (21.1136, 2.2, 3.0042) (12.8561, 2.2, 1.7678) (16.3916, 2.2, -1.7678) (18.1094, 2.2, -3.5355) (21.1136, 2.2, -7.6024) (21.1136, 2.2, -3.0042) (21.1136, 2.2, 7.6024) (18.1094, 2.2, -7.0711) (11.0883, 2.2, -7.0711) (7.5528, 2.2, -3.5355) (2.2495, 2.2, -8.8388) (-3.0538, 2.2, -14.1421) (-4.8216, 2.2, -12.3744) (-4.8216, 2.2, -8.8388) (-8.3571, 2.2, -8.8388) (-8.3571, 2.2, -12.3744) (-10.1249, 2.2, -14.1421) (-13.6604, 2.2, -14.1421) (-13.6604, 2.2, -17.6777) (-10.1249, 2.2, -17.6777) (-15.4282, 2.2, -19.4454) (16.3916, 2.2, -8.8388) (16.3916, 2.2, -12.3744) (18.1094, 2.2, -14.1421) (21.1136, 2.2, -13.6108) (21.1136, 2.2, -18.209) (18.1094, 2.2, -17.6777) (12.8561, 2.2, -12.3744) (12.8561, 2.2, -8.8388) (11.0883, 2.2, -14.1421) (7.5528, 2.2, -14.1421) (7.5528, 2.2, -17.6777) (11.0883, 2.2, -17.6777) (5.785, 2.2, -19.4454) (2.2495, 2.2, -19.4454) (2.2495, 2.2, -22.981) (5.785, 2.2, -22.981) (0.4817, 2.2, -17.6777) (-4.8216, 2.2, -22.981) (5.785, 2.2, -12.3744) (-10.1249, 2.2, -28.2843) (-15.4282, 2.2, -33.5876) (-20.6318, 2.2, -38.6413) (-20.6318, 2.2, -35.205) (-18.9637, 2.2, -33.5876) (-15.4282, 2.2, -40.6586) (-18.9637, 2.2, -40.6586) (-13.6604, 2.2, -38.8909) (-10.1249, 2.2, -35.3553) (-8.3571, 2.2, -33.5876) (-4.8216, 2.2, -30.052) (-3.0538, 2.2, -28.2843) (0.4817, 2.2, -24.7487) (-8.3571, 2.2, -30.052) (-13.6604, 2.2, -35.3553) (-10.1249, 2.2, -38.8909) (-4.8216, 2.2, -33.5876) (0.4817, 2.2, -28.2843) (-3.0538, 2.2, -24.7487) (7.5528, 2.2, -24.7487) (12.8561, 2.2, -19.4454) (2.2495, 2.2, -30.052) (-3.0538, 2.2, -35.3553) (-8.3571, 2.2, -40.6586) (-4.8216, 2.2, -40.6586) (-3.0538, 2.2, -38.8909) (0.4817, 2.2, -35.3553) (2.2495, 2.2, -33.5876) (5.785, 2.2, -30.052) (7.5528, 2.2, -28.2843) (11.0883, 2.2, -24.7487) (12.8561, 2.2, -22.981) (16.3916, 2.2, -19.4454) (21.1136, 2.2, -24.2174) (18.1094, 2.2, -28.2843) (16.3916, 2.2, -30.052) (12.8561, 2.2, -33.5876) (11.0883, 2.2, -35.3553) (7.5528, 2.2, -38.8909) (5.785, 2.2, -40.6586) (18.1094, 2.2, -24.7487) (16.3916, 2.2, -22.981) (11.0883, 2.2, -28.2843) (12.8561, 2.2, -30.052) (5.785, 2.2, -33.5876) (7.5528, 2.2, -35.3553) (0.4817, 2.2, -38.8909) (2.2495, 2.2, -40.6586) (18.1094, 2.2, -35.3553) (16.3916, 2.2, -33.5876) (21.1136, 2.2, -28.8156) (21.1136, 2.2, -34.824) (18.1094, 2.2, -38.8909) (16.3916, 2.2, -40.6586) (21.1136, 2.2, -39.4222) (11.0883, 2.2, -38.8909) (12.8561, 2.2, -40.6586) (-20.6318, 2.2, -56.4182) (-19.6955, 2.2, -58.9182) (-18.9637, 2.2, -54.8008) (-18.9637, 2.2, -51.2652) (-20.6318, 2.2, -49.2479) (-15.4282, 2.2, -54.8008) (-13.6604, 2.2, -56.3685) (-14.6463, 2.2, -58.9182) (-10.1249, 2.2, -56.3685) (-9.1389, 2.2, -58.9182) (-13.6604, 2.2, -49.4975) (-15.4282, 2.2, -51.2652) (-18.9637, 2.2, -44.1942) (-20.6318, 2.2, -45.8116) (-15.4282, 2.2, -44.1942) (-13.6604, 2.2, -45.9619) (-10.1249, 2.2, -49.4975) (-8.3571, 2.2, -51.2652) (-4.8216, 2.2, -54.8008) (-3.0538, 2.2, -56.3685) (5.785, 2.2, -44.1942) (7.5528, 2.2, -45.9619) (11.0883, 2.2, -49.4975) (12.8561, 2.2, -51.2652) (16.3916, 2.2, -54.8008) (18.0969, 2.2, -56.431) (21.0761, 2.2, -55.9997) (21.1136, 2.2, -50.0288) (21.1136, 2.2, -45.4306) (18.1094, 2.2, -45.9619) (18.1094, 2.2, -49.4975) (12.8561, 2.2, -44.1942) (16.3916, 2.2, -44.1942) (5.785, 2.2, -51.2652) (2.2495, 2.2, -54.8008) (0.4817, 2.2, -56.3685) (-4.0397, 2.2, -58.9182) (1.4677, 2.2, -58.9182) (0.4817, 2.2, -49.4975) (-3.0538, 2.2, -49.4975) (-3.0538, 2.2, -45.9619) (0.4817, 2.2, -45.9619) (2.2495, 2.2, -44.1942) (11.0883, 2.2, -56.3685) (6.5669, 2.2, -58.9182) (7.5528, 2.2, -56.3685) (12.0743, 2.2, -58.9182) (5.785, 2.2, -54.8008) (2.2495, 2.2, -51.2652) (7.5528, 2.2, -49.4975) (11.0883, 2.2, -45.9619) (12.8561, 2.2, -54.8008) (16.3916, 2.2, -51.2652) (17.1735, 2.2, -58.9182) (-10.1249, 2.2, -45.9619) (-8.3571, 2.2, -44.1942) (-4.8216, 2.2, -44.1942)
fillet "Fillet1" radius 1 4 edges at (27.35, 2.2, 0) (0, 2.2, 64.7) (0, 2.2, -64.7) (-27.35, 2.2, 0)
body "Solid1"
